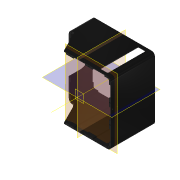
# Autodesk Inventor part: 30_XYTabel_Aliexpress_naked_splithousing
Saved by Autodesk Inventor 2022 (Build 260153000, 153)
## iProperties
Created: 2021-11-18
Part Number: 30_XYTabel_Aliexpress_naked_splithousing
Material: Generic
Document SubType Name: Modeling
Designer: diederichbenedict
Density: 1 g/cm^3
Appearance: Glatt - Schwarz
Mass: 169.721 g
Surface Area: 1363.63 cm^2
Volume: 169.721 cm^3
Author: diederichbenedict
Autodesk Inventor part; units mm, degrees
ref_plane "YZ Plane" through (0, 0, 0) normal (1, 0, 0) x (0, 1, 0)
ref_plane "XZ Plane" through (0, 0, 0) normal (0, 1, 0) x (-1, 0, 0)
ref_plane "XY Plane" through (0, 0, 0) normal (0, 0, 1) x (1, 0, 0)
ref_plane "Arbeitsebene18" through (-71.9552, 40.2052, -7) normal (0, 0, -1) x (-1, 0, 0)
sketch "Skizze14" plane through (-71.9552, 40.2052, -7) normal (0, 0, -1) x (-1, 0, 0)
  line L0 (73.5, 77.5) -> (-73.5, 77.5)
  line L1 (-77.5, 73.5) -> (-77.5, -73.5)
  line L2 (-73.5, -77.5) -> (73.5, -77.5)
  line L3 (77.5, -73.5) -> (77.5, 73.5)
  line L4 (77.5, 77.5) -> (-77.5, -77.5) construction
  line L5 (-77.5, 77.5) -> (77.5, -77.5) construction
  arc A0 (-77.5, -73.5) -> (-73.5, -77.5) centre (-73.5, -73.5) ccw
  arc A1 (-73.5, 77.5) -> (-77.5, 73.5) centre (-73.5, 73.5) ccw
  arc A2 (77.5, 73.5) -> (73.5, 77.5) centre (73.5, 73.5) ccw
  arc A3 (73.5, -77.5) -> (77.5, -73.5) centre (73.5, -73.5) ccw
  line L6 (-82.5, -73.5) -> (-82.5, 73.5)
  arc A4 (-73.5, 82.5) -> (-82.5, 73.5) centre (-73.5, 73.5) ccw
  line L7 (-73.5, 82.5) -> (73.5, 82.5)
  arc A5 (82.5, 73.5) -> (73.5, 82.5) centre (73.5, 73.5) ccw
  line L8 (82.5, 73.5) -> (82.5, -73.5)
  arc A6 (73.5, -82.5) -> (82.5, -73.5) centre (73.5, -73.5) ccw
  line L9 (73.5, -82.5) -> (-73.5, -82.5)
  arc A7 (-82.5, -73.5) -> (-73.5, -82.5) centre (-73.5, -73.5) ccw
  point P0 (0, 0)
  dimension "d192" = 155
  dimension "d193" = 155
  dimension "d196" = 165
  dimension "d210" = 4
  constraints: 20 end point, 16 point on circle, 8 centre point, 8 point on line, 8 tangent, 4 parallel, 3 equal radius, 3 midpoint, 2 perpendicular, 1 horizontal, 7 other
  measures "d192" distance of L5.end L4.end
  measures "d193" distance of L4.end L5.start
  measures "d196" distance between parallel lines of L7 L9
  measures "d210" radius of A2
extrude "Extrusion7" add sketch "Skizze14" along normal blind 115
ref_plane "Arbeitsebene19" through (-145.4552, 40.2052, -7) normal (0, -1, 0) x (1, 0, 0)
ref_plane "Arbeitsebene20" through (-71.9552, -33.2948, -7) normal (1, 0, 0) x (0, 0, -1)
sketch "Skizze27" plane through (-145.4552, 122.7052, -7) normal (0, 1, 0) x (1, 0, 0)
  line L0 (33, -6) -> (33, 0) projected
  line L1 (33, 0) -> (5.332, 55)
  line L2 (5.332, 55) -> (-9, 55)
  line L3 (0, 0) -> (147, 0) projected
  line L4 (-9, 0) -> (-9, 115) projected
  line L5 (-9, 55) -> (-9, 0)
  line L6 (-9, 0) -> (33, 0)
  point P0 (145.4552, -7)
  point P1 (-9, 55)
  dimension "d197" = 55
  constraints: 8 end point, 1 parallel, 1 perpendicular, 1 vertical
  measures "d197" distance between parallel lines of L2 L3
extrude "Extrusion15" cut sketch "Skizze27" against normal through all
sketch "Skizze28" plane through (-71.9552, 40.2052, -122) normal (0, 0, -1) x (-1, 0, 0)
  line L0 (-77.5, -73.5) -> (-77.5, 73.5) projected
  line L1 (-74.5, 15) -> (-80.5, 15)
  line L2 (-80.5, 15) -> (-80.5, -15)
  line L3 (-80.5, -15) -> (-74.5, -15)
  line L4 (-74.5, -15) -> (-74.5, 15)
  line L5 (-77.5, -73.5) -> (-77.5, 73.5) projected
  line L6 (-74.5, 15) -> (-80.5, -15) construction
  line L7 (-80.5, 15) -> (-74.5, -15) construction
  line L8 (-82.5, 73.5) -> (-82.5, -73.5) projected
  line L9 (-82.5, 73.5) -> (-82.5, 25.9699) projected
  circle A0 centre (-80, 25) radius 1.6
  circle A1 centre (-80, -25) radius 1.6
  point P0 (-71.9552, -40.2052)
  point P1 (-77.5, 0)
  point P2 (-77.5, -15)
  point P3 (-77.5, 15)
  dimension "d200" = 30
  dimension "d201" = 2
  dimension "d211" = 3.2
  dimension "d212" = 2.5
  dimension "d213" = 25
  dimension "d214" = 3.2
  dimension "d215" = 25
  constraints: 12 end point, 3 midpoint, 2 centre point, 2 parallel, 1 horizontal, 1 perpendicular
  measures "d200" distance of L2.end L1.end
  measures "d201" distance between parallel lines of L8 L2
  measures "d211" diameter of A0
  measures "d212" distance from line of A0.centre L8
  measures "d213" vertical distance of A0.centre point (-77.5, 0)
  measures "d214" diameter of A1
  measures "d215" vertical distance of A1.centre point (-77.5, 0)
extrude "Extrusion16" cut sketch "Skizze28" against normal through all
pattern_linear "Rechteckige Anordnung3" count 3 spacing 50 along (0, 1, 0) of "Extrusion16" first direction both ways yes
pattern_circular "Runde Anordnung3" count 4 over 360 about axis through (-71.9552, 40.2052, -7) along (0, 0, 1) of "Extrusion16", "Rechteckige Anordnung3"
sketch "Skizze31" plane through (-145.4552, 122.7052, -122) normal (0, 1, 0) x (1, 0, 0)
  circle A0 centre (63.8787, -99) radius 3.25 projected
  circle A1 centre (83.1213, -111.1914) radius 3.25 projected
  circle A2 centre (83.1213, -99) radius 3.25 projected
  circle A3 centre (63.8787, -111.1914) radius 3.25 projected
  line L0 (91.1213, -119.1914) -> (55.8787, -119.1914) projected
  line L1 (91.1213, -91) -> (91.1213, -119.1914) projected
  line L2 (81.2186, -91) -> (91.1213, -91) projected
  line L3 (55.8787, -119.1914) -> (55.8787, -91) projected
  arc A4 (67.7814, -93) -> (65.7814, -91) centre (65.7814, -93) ccw projected
  arc A5 (81.2186, -91) -> (79.2186, -93) centre (81.2186, -93) ccw projected
  line L4 (79.2186, -93) -> (79.2186, -102.798) projected
  arc A6 (67.7814, -102.798) -> (79.2186, -102.798) centre (73.5, -102.798) ccw projected
  line L5 (67.7814, -102.798) -> (67.7814, -93) projected
  line L6 (55.8787, -91) -> (65.7814, -91) projected
  point P0 (145.4552, -122)
hole "Bohrung9" at (-62.334, 122.7052, -10.8086) at (-81.5765, 122.7052, -10.8086) at (-62.334, 122.7052, -23) at (-81.5765, 122.7052, -23) direction (0, -1, 0) diameter 2.8 end through all
sketch "Skizze32" plane through (-154.4552, -42.2948, -122) normal (-1, 0, 0) x (0, -1, 0)
  line L0 (73.5, 124) -> (73.5, 110)
  circle A0 centre (-82.5, 30) radius 23.0002
  line L1 (-105.5, 30.0973) -> (-59.5, 30.0973)
  line L2 (-59.5, 30.0973) -> (-59.5, 73.6062)
  line L3 (-59.5, 73.6062) -> (-105.5, 73.6062)
  line L4 (-105.5, 73.6062) -> (-105.5, 30.0973)
  line L5 (-165, 60) -> (-165, 0) projected
  line L6 (0, 60) -> (0, 0) projected
  line L7 (-9, 0) -> (-156, 0) projected
  point P0 (-42.2948, 122)
  point P1 (-59.5, 30.0973)
  dimension "d243" = 165
  dimension "d244" = 82.5
  dimension "d245" = 30
  constraints: 10 end point, 2 parallel, 1 horizontal, 1 perpendicular, 1 vertical, 5 other
  measures "d243" distance between parallel lines of L6 L5
  measures "d244" distance from line of point (-82.5, 30) L5
  measures "d245" distance from line of L7 point (-82.5, 30)
extrude "Extrusion19" cut sketch "Skizze32" against normal blind 10
sketch "Skizze33" plane through (1.5448, 117.7052, -122) normal (0, -1, 0) x (1, 0, 0)
  line L0 (-6.5, 8) -> (-26.5, 8)
  line L1 (-26.5, 8) -> (-26.5, 108)
  line L2 (-26.5, 108) -> (-6.5, 108)
  line L3 (-6.5, 108) -> (-6.5, 8)
  line L4 (9, 115) -> (9, 0) projected
  point P0 (-1.5448, 122)
  point P1 (-8.075, 108)
  point P2 (-8.075, 8.6)
  point P3 (-6.5, 8.6)
  dimension "d238" = 100
  dimension "d239" = 20
  dimension "d240" = 0
  dimension "d241" = 0
  dimension "d289" = 15.5
  constraints: 8 end point, 2 parallel, 1 horizontal, 1 perpendicular, 4 other
  measures "d238" distance between parallel lines of L0 L2
  measures "d239" distance between parallel lines of L1 L3
  measures "d240" distance of point (-6.5, 108) L2.end
  measures "d241" distance from line of L3 point (-6.5, 108)
  measures "d289" distance between parallel lines of L3 L4
extrude "Extrusion20" cut sketch "Skizze33" against normal blind 10
fillet "Rundung3" radius 2 4 edges at (-24.9552, 121.7052, -14) (-4.9552, 120.2052, -14) (-4.9552, 120.2052, -114) (-24.9552, 121.7052, -114)
ref_plane "Arbeitsebene21" through (-71.9552, 40.2052, -17) normal (0, 0, 1) x (1, 0, 0)
sketch "Skizze35" plane through (-140.1232, 117.7052, -62) normal (-0.8933333, 0, 0.4493947) x (0.4493947, 0, 0.8933333)
  ellipse E0 centre (56.7281, 1) end of major axis (56.7281, -0.4) minor radius 1.3801 projected
  ellipse E1 centre (56.7281, -156) end of major axis (56.7281, -157.4) minor radius 1.3801 projected
  point P0 (118.3573, -117.7052)
extrude "Extrusion22" cut sketch "Skizze35" against normal blind 20
pattern_circular "Runde Anordnung4" count 2 over 90 about axis through (-71.9552, 40.2052, 0) along (0, 0, 1) of "Bohrung9"
